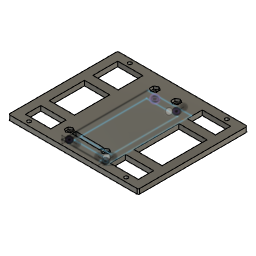
EmlaSafe - Adapter Plate (Autodesk Fusion 360 design; units mm, degrees)
Autodesk Fusion 360 part; units mm, degrees
(part 1 of 2)
sketch "Sketch1" plane through (0, 0, 0) normal (0, 0, 1) x (1, 0, 0)
  line L0 (15.5775, 37.2124) -> (15.5775, 44.1528) construction
  circle A0 centre (15.5775, 40.6826) radius 3.5
  line L1 (33.2439, 37.2427) -> (33.2439, 44.2427) construction
  circle A1 centre (33.2439, 40.7427) radius 3.5
  circle A2 centre (6.7, -23.6) radius 1.65
  circle A3 centre (42.4985, -23.8668) radius 1.65
  line L2 (6.7, -23.6) -> (6.7, -21.95) construction
  line L3 (6.7, -23.6) -> (6.7, -25.25) construction
  line L4 (42.4985, -23.8668) -> (42.4985, -22.2168) construction
  line L5 (42.4985, -23.8668) -> (42.4985, -25.5168) construction
  line L6 (42.4985, -22.2168) -> (35.9985, -22.2168)
  line L7 (35.9985, -22.2168) -> (35.9985, -25.4858)
  line L8 (35.9985, -25.4858) -> (42.4985, -25.4858)
  line L9 (42.4985, -25.4858) -> (42.4985, -22.2168)
  line L10 (6.7, -25.25) -> (13.2, -25.25)
  line L11 (13.2, -25.25) -> (13.2, -21.981)
  line L12 (13.2, -21.981) -> (6.7, -21.981)
  line L13 (6.7, -21.981) -> (6.7, -25.25)
  line L14 (50, 45) -> (50, -29)
  line L15 (50, -29) -> (1, -29)
  line L16 (1, -29) -> (1, 45)
  line L17 (13.2, -21.981) -> (35.9985, -22.2168)
  line L18 (35.9985, -25.4858) -> (13.2, -25.25)
  line L19 (50, 45) -> (50, 46.2)
  line L20 (50, 46.2) -> (1, 46.2)
  line L21 (1, 46.2) -> (1, 45)
  line L22 (8, 33) -> (8, -18)
  line L23 (43, 33) -> (43, -18)
  line L24 (43, -18) -> (8, -18)
  line L25 (8, 33) -> (43, 33)
  dimension "d1" = 7
  dimension "d2" = 7
  dimension "d3" = 3.3
  dimension "d4" = 3.3
  dimension "d5" = 6.5
  dimension "d6" = 6.5
  dimension "d7" = 49
  dimension "d8" = 74
  dimension "d15" = 1.2
  constraint vertical L0
  constraint midpoint L0 A0.centre
  constraint vertical L1
  constraint midpoint L1 A1.centre
  constraint coincident A2.centre L2.start
  constraint coincident A2 L2.end
  constraint vertical L2
  constraint coincident A2 L3.end
  constraint parallel L2 L3
  constraint coincident A3.centre L4.start
  constraint coincident A3 L4.end
  constraint vertical L4
  constraint coincident A3 L5.end
  constraint parallel L4 L5
  constraint horizontal L6
  constraint vertical L7
  constraint horizontal L8
  constraint vertical L9
  constraint horizontal L10
  constraint vertical L11
  constraint horizontal L12
  constraint vertical L13
  constraint vertical L14
  constraint horizontal L15
  constraint vertical L16
  constraint parallel L17 L18
  constraint vertical L19
  constraint horizontal L20
  constraint vertical L21
  constraint perpendicular L23 L24
  measures "d1" diameter of A1
  measures "d2" diameter of A0
  measures "d3" diameter of A2
  measures "d4" diameter of A3
  measures "d5" distance of L4.end L6.end
  measures "d6" distance of L3.end L10.end
  measures "d7" distance of L14.end L15.end
  measures "d8" distance of L14.start L14.end
  measures "d15" distance of L16.end L20.end
extrude "Extrude1" add sketch "Sketch1" along normal blind 1 contours L14 L15 L16 L19 L20 L21 | L22 L23 L24 L25 makes body 1
extrude "Extrude2" add sketch "Sketch1" along normal blind -3 and the other way blind -1 contours A0 | A1 | A2 L12 L13 | A2 L10 L11 L12 | A2 L12 L13 | A3 L6 L7 L8 | A3 L8 L9 | A3 L8 L9 bodies 1
sketch "Sketch2" plane through (0, 0, 0) normal (0, 0, 1) x (1, 0, 0)
  line L0 (79.2304, 52.3866) -> (-25.7696, 52.3866)
  line L1 (-9.7696, 51.3866) -> (63.2304, 51.3866)
  line L2 (-25.7696, -37.6134) -> (79.2304, -37.6134)
  line L3 (63.2304, -36.6134) -> (-9.7696, -36.6134)
  line L4 (-10.892, -33.3408) -> (-10.9857, -33.0965)
  line L5 (65.0576, -32.2555) -> (64.8725, -32.4405)
  line L6 (64.2304, 48.8866) -> (64.2441, 48.6253)
  line L7 (-10.9857, -33.0965) -> (-11.1045, -32.8634)
  line L8 (80.2085, -36.8213) -> (80.2304, -36.6134)
  line L9 (64.8725, -32.4405) -> (64.7079, -32.6439)
  line L10 (64.7079, -32.6439) -> (64.5653, -32.8634)
  line L11 (65.7538, -34.3283) -> (65.7304, -34.1134)
  line L12 (79.2249, -30.7179) -> (79.1814, -30.9224)
  line L13 (65.9579, 46.509) -> (66.2106, 46.4413)
  line L14 (66.1692, -33.2857) -> (66.3603, -33.1844)
  line L15 (79.2304, -30.6134) -> (79.2249, -30.7179)
  line L16 (66.4691, -31.6271) -> (66.2106, -31.668)
  line L17 (79.0964, -31.1134) -> (78.9735, -31.2825)
  line L18 (79.1814, -30.9224) -> (79.0964, -31.1134)
  line L19 (66.3603, -33.1844) -> (66.5686, -33.1265)
  line L20 (65.7304, -34.1134) -> (65.7363, -34.0052)
  line L21 (66.2106, 46.4413) -> (66.4691, 46.4003)
  line L22 (66.2106, -31.668) -> (65.9579, -31.7357)
  line L23 (79.2304, -37.6134) -> (79.3349, -37.6079)
  line L24 (67.2916, -33.2857) -> (67.3778, -33.3512)
  line L25 (67.1988, -33.2298) -> (67.2916, -33.2857)
  line L26 (-11.8001, 46.8641) -> (-11.5968, 47.0288)
  line L27 (65.9343, 48.2815) -> (65.8228, 48.4668)
  line L28 (66.083, 48.1245) -> (65.9343, 48.2815)
  line L29 (67.3778, -33.3512) -> (67.5265, -33.5082)
  line L30 (79.3349, -37.6079) -> (79.5394, -37.5644)
  line L31 (64.2304, -34.1134) -> (64.2304, -35.6134)
  line L32 (-11.5968, 47.0288) -> (-11.4117, 47.2138)
  line L33 (64.2304, -35.6134) -> (64.2085, -35.8213)
  line L34 (-12.2528, -31.8295) -> (-12.4971, -31.7357)
  line L35 (-12.0196, -31.9483) -> (-12.2528, -31.8295)
  line L36 (65.7538, 48.6717) -> (65.7304, 48.8866)
  line L37 (66.7845, -33.1148) -> (66.9979, -33.1498)
  line L38 (-12.6222, -33.3512) -> (-12.4735, -33.5082)
  line L39 (64.2441, -33.852) -> (64.2304, -34.1134)
  line L40 (66.5686, -33.1265) -> (66.7845, -33.1148)
  line L41 (66.9979, -33.1498) -> (67.1988, -33.2298)
  line L42 (78.6371, -31.5269) -> (78.4383, -31.5915)
  line L43 (78.9735, -31.2825) -> (78.8182, -31.4224)
  line L44 (65.8228, 48.4668) -> (65.7538, 48.6717)
  line L45 (-12.4971, 46.509) -> (-12.2528, 46.6028)
  line L46 (-12.362, -33.6935) -> (-12.293, -33.8984)
  line L47 (78.8182, -31.4224) -> (78.6371, -31.5269)
  line L48 (-12.2528, 46.6028) -> (-12.0196, 46.7216)
  line L49 (78.4383, -31.5915) -> (78.2304, -31.6134)
  line L50 (-12.0196, 46.7216) -> (-11.8001, 46.8641)
  line L51 (-12.4735, -33.5082) -> (-12.362, -33.6935)
  line L52 (-12.362, 48.4668) -> (-12.4735, 48.2815)
  line L53 (80.0394, -37.2011) -> (80.1439, -37.0201)
  line L54 (-11.2471, -32.6439) -> (-11.4117, -32.4405)
  line L55 (64.3528, 48.1141) -> (64.4465, 47.8698)
  line L56 (79.8995, -37.3565) -> (80.0394, -37.2011)
  line L57 (65.7136, -31.8295) -> (65.4804, -31.9483)
  line L58 (-11.4117, -32.4405) -> (-11.5968, -32.2555)
  line L59 (65.9579, -31.7357) -> (65.7136, -31.8295)
  line L60 (-12.293, 48.6717) -> (-12.362, 48.4668)
  line L61 (64.4465, 47.8698) -> (64.5653, 47.6366)
  line L62 (78.2304, -31.6134) -> (66.7304, -31.6134)
  line L63 (-24.7696, 46.3866) -> (-13.2696, 46.3866)
  line L64 (64.4465, -33.0965) -> (64.3528, -33.3408)
  line L65 (64.5653, -32.8634) -> (64.4465, -33.0965)
  line L66 (-10.7833, -33.852) -> (-10.8242, -33.5936)
  line L67 (-10.8242, -33.5936) -> (-10.892, -33.3408)
  line L68 (80.1439, -37.0201) -> (80.2085, -36.8213)
  line L69 (-12.2696, 48.8866) -> (-12.293, 48.6717)
  line L70 (64.285, 48.3669) -> (64.3528, 48.1141)
  line L71 (-12.4735, 48.2815) -> (-12.6222, 48.1245)
  line L72 (-11.1045, -32.8634) -> (-11.2471, -32.6439)
  line L73 (65.2609, -32.0908) -> (65.0576, -32.2555)
  line L74 (65.4804, -31.9483) -> (65.2609, -32.0908)
  line L75 (64.2441, 48.6253) -> (64.285, 48.3669)
  line L76 (-12.6222, 48.1245) -> (-12.7084, 48.059)
  line L77 (-13.3237, 47.8881) -> (-13.5371, 47.9231)
  line L78 (-13.8308, -33.2857) -> (-13.6397, -33.1844)
  line L79 (-13.6397, -33.1844) -> (-13.4314, -33.1265)
  line L80 (66.262, 48.0031) -> (66.083, 48.1245)
  line L81 (-10.2696, -36.4794) -> (-10.4387, -36.3565)
  line L82 (-13.4314, -33.1265) -> (-13.2155, -33.1148)
  line L83 (-12.8995, 47.9577) -> (-13.1078, 47.8998)
  line L84 (-24.8741, -31.6079) -> (-25.0786, -31.5644)
  line L85 (67.2916, -34.941) -> (67.1005, -35.0423)
  line L86 (66.4629, -35.0769) -> (66.262, -34.9969)
  line L87 (-10.0786, -36.5644) -> (-10.2696, -36.4794)
  line L88 (-13.1078, 47.8998) -> (-13.3237, 47.8881)
  line L89 (66.8922, -35.1002) -> (66.6763, -35.1119)
  line L90 (-13.2155, -33.1148) -> (-13.0021, -33.1498)
  line L91 (-13.0021, -33.1498) -> (-12.8012, -33.2298)
  line L92 (66.8922, 47.8998) -> (66.6763, 47.8881)
  line L93 (-24.7696, -31.6134) -> (-24.8741, -31.6079)
  line L94 (-13.9956, -33.4257) -> (-13.8308, -33.2857)
  line L95 (66.6763, 47.8881) -> (66.4629, 47.9231)
  line L96 (66.4629, 47.9231) -> (66.262, 48.0031)
  line L97 (-9.7696, -36.6134) -> (-9.8741, -36.6079)
  line L98 (-9.8741, -36.6079) -> (-10.0786, -36.5644)
  line L99 (67.1005, -35.0423) -> (66.8922, -35.1002)
  line L100 (-12.7084, 48.059) -> (-12.8995, 47.9577)
  line L101 (66.6763, -35.1119) -> (66.4629, -35.0769)
  line L102 (-14.2173, -33.7941) -> (-14.1265, -33.5978)
  line L103 (-12.7498, -31.668) -> (-13.0083, -31.6271)
  line L104 (67.707, 48.6717) -> (67.638, 48.4668)
  line L105 (-14.0657, 48.2815) -> (-14.1772, 48.4668)
  line L106 (66.262, -34.9969) -> (66.083, -34.8755)
  line L107 (-13.2696, -31.6134) -> (-24.7696, -31.6134)
  line L108 (-14.1265, -33.5978) -> (-13.9956, -33.4257)
  line L109 (-12.4971, -31.7357) -> (-12.7498, -31.668)
  line L110 (-13.0083, -31.6271) -> (-13.2696, -31.6134)
  line L111 (-13.917, 48.1245) -> (-14.0657, 48.2815)
  line L112 (66.7304, -31.6134) -> (66.4691, -31.6271)
  line L113 (67.7304, 48.8866) -> (67.707, 48.6717)
  line L114 (67.3778, 48.1245) -> (67.2916, 48.059)
  line L115 (67.2916, 48.059) -> (67.1005, 47.9577)
  line L116 (66.083, -34.8755) -> (65.9343, -34.7185)
  line L117 (66.4691, 46.4003) -> (66.7304, 46.3866)
  line L118 (65.8228, -34.5333) -> (65.7538, -34.3283)
  line L119 (66.7304, 46.3866) -> (78.2304, 46.3866)
  line L120 (-14.2462, 48.6717) -> (-14.2696, 48.8866)
  line L121 (67.1005, 47.9577) -> (66.8922, 47.8998)
  line L122 (-14.2637, -34.0052) -> (-14.2173, -33.7941)
  line L123 (67.5265, 48.2815) -> (67.3778, 48.1245)
  line L124 (-13.5371, 47.9231) -> (-13.738, 48.0031)
  line L125 (67.638, 48.4668) -> (67.5265, 48.2815)
  line L126 (-13.738, 48.0031) -> (-13.917, 48.1245)
  line L127 (65.9343, -34.7185) -> (65.8228, -34.5333)
  line L128 (-14.1772, 48.4668) -> (-14.2462, 48.6717)
  line L129 (-12.8995, -35.0423) -> (-13.1078, -35.1002)
  line L130 (-12.7084, -34.941) -> (-12.8995, -35.0423)
  line L131 (66.1692, 49.7143) -> (66.3603, 49.8156)
  line L132 (78.4383, 46.3648) -> (78.6371, 46.3002)
  line L133 (78.6371, 46.3002) -> (78.8182, 46.1957)
  line L134 (-10.7207, 50.6957) -> (-10.6356, 50.8866)
  line L135 (-13.1078, -35.1002) -> (-13.3237, -35.1119)
  line L136 (78.9735, 46.0558) -> (79.0964, 45.8866)
  line L137 (-13.3237, -35.1119) -> (-13.5371, -35.0769)
  line L138 (66.5686, 49.8735) -> (66.7845, 49.8852)
  line L139 (-13.5371, -35.0769) -> (-13.738, -34.9969)
  line L140 (66.7845, 49.8852) -> (66.9979, 49.8502)
  line L141 (66.3603, 49.8156) -> (66.5686, 49.8735)
  line L142 (66.0044, 49.5743) -> (66.1692, 49.7143)
  line L143 (-10.6356, 50.8866) -> (-10.5127, 51.0558)
  line L144 (-12.6222, 49.6488) -> (-12.4735, 49.4918)
  line L145 (79.1814, 45.6957) -> (79.2249, 45.4912)
  line L146 (-12.4735, 49.4918) -> (-12.362, 49.3065)
  line L147 (-12.7084, 49.7143) -> (-12.6222, 49.6488)
  line L148 (65.8735, 49.4022) -> (66.0044, 49.5743)
  line L149 (-12.293, 49.1016) -> (-12.2696, 48.8866)
  line L150 (66.9979, 49.8502) -> (67.1988, 49.7702)
  line L151 (-13.738, -34.9969) -> (-13.917, -34.8755)
  line L152 (79.2249, 45.4912) -> (79.2304, 45.3866)
  line L153 (78.8182, 46.1957) -> (78.9735, 46.0558)
  line L154 (-12.362, 49.3065) -> (-12.293, 49.1016)
  line L155 (67.1988, 49.7702) -> (67.2916, 49.7143)
  line L156 (79.0964, 45.8866) -> (79.1814, 45.6957)
  line L157 (-13.917, -34.8755) -> (-14.0657, -34.7185)
  line L158 (-12.8012, 49.7702) -> (-12.7084, 49.7143)
  line L159 (-26.7478, 51.5946) -> (-26.7696, 51.3866)
  line L160 (-10.7641, 50.4912) -> (-10.7207, 50.6957)
  line L161 (-14.0657, -34.7185) -> (-14.1772, -34.5333)
  line L162 (-14.2696, 48.8866) -> (-14.2637, 48.9948)
  line L163 (67.2916, 49.7143) -> (67.3778, 49.6488)
  line L164 (67.3778, 49.6488) -> (67.5265, 49.4918)
  line L165 (-14.1772, -34.5333) -> (-14.2462, -34.3283)
  line L166 (-13.0021, 49.8502) -> (-12.8012, 49.7702)
  line L167 (80.2304, 51.3866) -> (80.2085, 51.5946)
  line L168 (-10.7696, 48.8866) -> (-10.7696, 50.3866)
  line L169 (67.638, 49.3065) -> (67.707, 49.1016)
  line L170 (-26.2696, 52.2527) -> (-26.4387, 52.1298)
  line L171 (79.8995, 52.1298) -> (79.7304, 52.2527)
  line L172 (-13.8308, 49.7143) -> (-13.6397, 49.8156)
  line L173 (-25.7696, 45.3866) -> (-25.7478, 45.5946)
  line L174 (67.707, 49.1016) -> (67.7304, 48.8866)
  line L175 (-10.7696, 50.3866) -> (-10.7641, 50.4912)
  line L176 (80.2085, 51.5946) -> (80.1439, 51.7934)
  line L177 (-26.5786, 51.9744) -> (-26.6831, 51.7934)
  line L178 (67.5265, 49.4918) -> (67.638, 49.3065)
  line L179 (-13.2155, 49.8852) -> (-13.0021, 49.8502)
  line L180 (-26.4387, 52.1298) -> (-26.5786, 51.9744)
  line L181 (80.0394, 51.9744) -> (79.8995, 52.1298)
  line L182 (-13.6397, 49.8156) -> (-13.4314, 49.8735)
  line L183 (80.1439, 51.7934) -> (80.0394, 51.9744)
  line L184 (-26.6831, 51.7934) -> (-26.7478, 51.5946)
  line L185 (-13.4314, 49.8735) -> (-13.2155, 49.8852)
  line L186 (-14.2462, -34.3283) -> (-14.2696, -34.1134)
  line L187 (79.3349, 52.3812) -> (79.2304, 52.3866)
  line L188 (-10.8242, 48.3669) -> (-10.7833, 48.6253)
  line L189 (64.7079, 47.4172) -> (64.8725, 47.2138)
  line L190 (63.3349, -36.6079) -> (63.2304, -36.6134)
  line L191 (-10.7833, 48.6253) -> (-10.7696, 48.8866)
  line L192 (64.5653, 47.6366) -> (64.7079, 47.4172)
  line L193 (-10.7696, -35.6134) -> (-10.7696, -34.1134)
  line L194 (-12.7498, 46.4413) -> (-12.4971, 46.509)
  line L195 (67.638, -34.5333) -> (67.5265, -34.7185)
  line L196 (67.7304, -34.1134) -> (67.707, -34.3283)
  line L197 (-25.0786, -31.5644) -> (-25.2696, -31.4794)
  line L198 (-10.4387, -36.3565) -> (-10.5786, -36.2011)
  line L199 (63.4383, 51.3648) -> (63.6371, 51.3002)
  line L200 (-25.5786, -31.2011) -> (-25.6831, -31.0201)
  line L201 (67.3778, -34.8755) -> (67.2916, -34.941)
  line L202 (-10.7696, -34.1134) -> (-10.7833, -33.852)
  line L203 (-25.7478, -30.8213) -> (-25.7696, -30.6134)
  line L204 (63.9735, 51.0558) -> (64.0964, 50.8866)
  line L205 (-26.0786, -37.5644) -> (-25.8741, -37.6079)
  line L206 (-12.8012, -33.2298) -> (-12.7084, -33.2857)
  line L207 (-13.2696, 46.3866) -> (-13.0083, 46.4003)
  line L208 (-13.0083, 46.4003) -> (-12.7498, 46.4413)
  line L209 (67.5265, -34.7185) -> (67.3778, -34.8755)
  line L210 (-25.8741, -37.6079) -> (-25.7696, -37.6134)
  line L211 (67.707, -34.3283) -> (67.638, -34.5333)
  line L212 (-25.2696, -31.4794) -> (-25.4387, -31.3565)
  line L213 (63.2304, 51.3866) -> (63.4383, 51.3648)
  line L214 (-10.5786, -36.2011) -> (-10.6831, -36.0201)
  line L215 (-25.4387, -31.3565) -> (-25.5786, -31.2011)
  line L216 (-10.6831, -36.0201) -> (-10.7478, -35.8213)
  line L217 (63.6371, 51.3002) -> (63.8182, 51.1957)
  line L218 (-10.7478, -35.8213) -> (-10.7696, -35.6134)
  line L219 (63.8182, 51.1957) -> (63.9735, 51.0558)
  line L220 (-12.7084, -33.2857) -> (-12.6222, -33.3512)
  line L221 (-25.6831, -31.0201) -> (-25.7478, -30.8213)
  line L222 (63.7304, -36.4794) -> (63.5394, -36.5644)
  line L223 (79.7304, -37.4794) -> (79.8995, -37.3565)
  line L224 (63.5394, -36.5644) -> (63.3349, -36.6079)
  line L225 (63.8995, -36.3565) -> (63.7304, -36.4794)
  line L226 (-10.892, 48.1141) -> (-10.8242, 48.3669)
  line L227 (64.8725, 47.2138) -> (65.0576, 47.0288)
  line L228 (-10.9857, 47.8698) -> (-10.892, 48.1141)
  line L229 (65.0576, 47.0288) -> (65.2609, 46.8641)
  line L230 (66.0044, -33.4257) -> (66.1692, -33.2857)
  line L231 (64.1439, -36.0201) -> (64.0394, -36.2011)
  line L232 (-11.5968, -32.2555) -> (-11.8001, -32.0908)
  line L233 (64.0394, -36.2011) -> (63.8995, -36.3565)
  line L234 (65.4804, 46.7216) -> (65.7136, 46.6028)
  line L235 (67.638, -33.6935) -> (67.707, -33.8984)
  line L236 (-11.1045, 47.6366) -> (-10.9857, 47.8698)
  line L237 (-11.4117, 47.2138) -> (-11.2471, 47.4172)
  line L238 (65.2609, 46.8641) -> (65.4804, 46.7216)
  line L239 (79.5394, -37.5644) -> (79.7304, -37.4794)
  line L240 (65.7136, 46.6028) -> (65.9579, 46.509)
  line L241 (67.5265, -33.5082) -> (67.638, -33.6935)
  line L242 (64.2085, -35.8213) -> (64.1439, -36.0201)
  line L243 (-11.2471, 47.4172) -> (-11.1045, 47.6366)
  line L244 (-11.8001, -32.0908) -> (-12.0196, -31.9483)
  line L245 (80.2304, -36.6134) -> (80.2304, 51.3866)
  line L246 (79.2304, 7.3866) -> (79.2304, -30.6134)
  line L247 (79.2304, 45.3866) -> (79.2304, 7.3866)
  line L248 (64.285, -33.5936) -> (64.2441, -33.852)
  line L249 (64.3528, -33.3408) -> (64.285, -33.5936)
  line L250 (65.7827, -33.7941) -> (65.8735, -33.5978)
  line L251 (65.8735, -33.5978) -> (66.0044, -33.4257)
  line L252 (-26.7696, 51.3866) -> (-26.7696, -36.6134)
  line L253 (-25.7696, -30.6134) -> (-25.7696, 45.3866)
  line L254 (65.7363, -34.0052) -> (65.7827, -33.7941)
  line L255 (-25.7696, 52.3866) -> (-25.8741, 52.3812)
  line L256 (-25.4387, 46.1298) -> (-25.2696, 46.2527)
  line L257 (-13.9956, 49.5743) -> (-13.8308, 49.7143)
  line L258 (-14.1265, 49.4022) -> (-13.9956, 49.5743)
  line L259 (-25.5786, 45.9744) -> (-25.4387, 46.1298)
  line L260 (-26.0786, 52.3377) -> (-26.2696, 52.2527)
  line L261 (-14.2637, 48.9948) -> (-14.2173, 49.2059)
  line L262 (-25.0786, 46.3377) -> (-24.8741, 46.3812)
  line L263 (-25.2696, 46.2527) -> (-25.0786, 46.3377)
  line L264 (-25.7478, 45.5946) -> (-25.6831, 45.7934)
  line L265 (-24.8741, 46.3812) -> (-24.7696, 46.3866)
  line L266 (79.7304, 52.2527) -> (79.5394, 52.3377)
  line L267 (-14.2173, 49.2059) -> (-14.1265, 49.4022)
  line L268 (-25.8741, 52.3812) -> (-26.0786, 52.3377)
  line L269 (79.5394, 52.3377) -> (79.3349, 52.3812)
  line L270 (-25.6831, 45.7934) -> (-25.5786, 45.9744)
  line L271 (-26.7478, -36.8213) -> (-26.6831, -37.0201)
  line L272 (-10.5127, 51.0558) -> (-10.3574, 51.1957)
  line L273 (65.7827, 49.2059) -> (65.8735, 49.4022)
  line L274 (-26.2696, -37.4794) -> (-26.0786, -37.5644)
  line L275 (-10.3574, 51.1957) -> (-10.1763, 51.3002)
  line L276 (-12.293, -34.3283) -> (-12.362, -34.5333)
  line L277 (-12.293, -33.8984) -> (-12.2696, -34.1134)
  line L278 (-26.4387, -37.3565) -> (-26.2696, -37.4794)
  line L279 (64.2249, 50.4912) -> (64.2304, 50.3866)
  line L280 (64.2304, 50.3866) -> (64.2304, 48.8866)
  line L281 (-26.5786, -37.2011) -> (-26.4387, -37.3565)
  line L282 (64.0964, 50.8866) -> (64.1815, 50.6957)
  line L283 (-9.9775, 51.3648) -> (-9.7696, 51.3866)
  line L284 (-26.6831, -37.0201) -> (-26.5786, -37.2011)
  line L285 (65.7363, 48.9948) -> (65.7827, 49.2059)
  line L286 (78.2304, 46.3866) -> (78.4383, 46.3648)
  line L287 (-14.2696, -34.1134) -> (-14.2637, -34.0052)
  line L288 (-10.1763, 51.3002) -> (-9.9775, 51.3648)
  line L289 (-26.7696, -36.6134) -> (-26.7478, -36.8213)
  line L290 (67.707, -33.8984) -> (67.7304, -34.1134)
  line L291 (-12.4735, -34.7185) -> (-12.6222, -34.8755)
  line L292 (64.1815, 50.6957) -> (64.2249, 50.4912)
  line L293 (-12.2696, -34.1134) -> (-12.293, -34.3283)
  line L294 (-12.362, -34.5333) -> (-12.4735, -34.7185)
  line L295 (65.7304, 48.8866) -> (65.7363, 48.9948)
  line L296 (-12.6222, -34.8755) -> (-12.7084, -34.941)
  line L297 (79.2304, 52.3866) -> (79.3349, 52.3812)
  line L298 (-25.7696, 52.3866) -> (79.2304, 52.3866)
  line L299 (79.3349, 52.3812) -> (79.5394, 52.3377)
  line L300 (80.0394, 51.9744) -> (80.1439, 51.7934)
  line L301 (79.3349, -37.6079) -> (79.2304, -37.6134)
  line L302 (79.5394, 52.3377) -> (79.7304, 52.2527)
  line L303 (79.8995, 52.1298) -> (80.0394, 51.9744)
  line L304 (-26.7696, -36.6134) -> (-26.7696, 51.3866)
  line L305 (79.5394, -37.5644) -> (79.3349, -37.6079)
  line L306 (79.8995, -37.3565) -> (79.7304, -37.4794)
  line L307 (-26.6831, -37.0201) -> (-26.7478, -36.8213)
  line L308 (79.7304, -37.4794) -> (79.5394, -37.5644)
  line L309 (80.1439, -37.0201) -> (80.0394, -37.2011)
  line L310 (80.2304, -36.6134) -> (80.2085, -36.8213)
  line L311 (80.2304, 51.3866) -> (80.2304, -36.6134)
  line L312 (80.0394, -37.2011) -> (79.8995, -37.3565)
  line L313 (-26.7696, 51.3866) -> (-26.7478, 51.5946)
  line L314 (80.1439, 51.7934) -> (80.2085, 51.5946)
  line L315 (79.2304, -37.6134) -> (-25.7696, -37.6134)
  line L316 (-25.8741, -37.6079) -> (-26.0786, -37.5644)
  line L317 (-25.7696, -37.6134) -> (-25.8741, -37.6079)
  line L318 (-26.2696, -37.4794) -> (-26.4387, -37.3565)
  line L319 (79.7304, 52.2527) -> (79.8995, 52.1298)
  line L320 (-26.7478, -36.8213) -> (-26.7696, -36.6134)
  line L321 (-26.0786, -37.5644) -> (-26.2696, -37.4794)
  line L322 (80.2085, -36.8213) -> (80.1439, -37.0201)
  line L323 (-13.2696, -31.6134) -> (-13.0083, -31.6271)
  line L324 (-9.7696, 51.3866) -> (-9.9775, 51.3648)
  line L325 (-10.7833, 48.6253) -> (-10.8242, 48.3669)
  line L326 (-10.7641, 50.4912) -> (-10.7696, 50.3866)
  line L327 (-25.2696, 46.2527) -> (-25.4387, 46.1298)
  line L328 (-11.8001, -32.0908) -> (-11.5968, -32.2555)
  line L329 (-25.4387, 46.1298) -> (-25.5786, 45.9744)
  line L330 (-25.0786, 46.3377) -> (-25.2696, 46.2527)
  line L331 (-9.9775, 51.3648) -> (-10.1763, 51.3002)
  line L332 (-10.5127, 51.0558) -> (-10.6356, 50.8866)
  line L333 (-25.7696, -30.6134) -> (-25.7478, -30.8213)
  line L334 (-25.5786, 45.9744) -> (-25.6831, 45.7934)
  line L335 (-11.5968, -32.2555) -> (-11.4117, -32.4405)
  line L336 (-11.2471, 47.4172) -> (-11.4117, 47.2138)
  line L337 (-11.4117, 47.2138) -> (-11.5968, 47.0288)
  line L338 (-12.0196, 46.7216) -> (-12.2528, 46.6028)
  line L339 (-10.6356, 50.8866) -> (-10.7207, 50.6957)
  line L340 (-13.0083, -31.6271) -> (-12.7498, -31.668)
  line L341 (-26.7478, 51.5946) -> (-26.6831, 51.7934)
  line L342 (-25.7478, -30.8213) -> (-25.6831, -31.0201)
  line L343 (-10.7696, 48.8866) -> (-10.7833, 48.6253)
  line L344 (-13.2696, 46.3866) -> (-24.7696, 46.3866)
  line L345 (-25.5786, -31.2011) -> (-25.4387, -31.3565)
  line L346 (-11.5968, 47.0288) -> (-11.8001, 46.8641)
  line L347 (-11.1045, 47.6366) -> (-11.2471, 47.4172)
  line L348 (-10.892, 48.1141) -> (-10.9857, 47.8698)
  line L349 (-12.2528, 46.6028) -> (-12.4971, 46.509)
  line L350 (-11.8001, 46.8641) -> (-12.0196, 46.7216)
  line L351 (-12.7498, -31.668) -> (-12.4971, -31.7357)
  line L352 (-26.5786, -37.2011) -> (-26.6831, -37.0201)
  line L353 (-12.0196, -31.9483) -> (-11.8001, -32.0908)
  line L354 (-10.7696, 50.3866) -> (-10.7696, 48.8866)
  line L355 (-11.2471, -32.6439) -> (-11.1045, -32.8634)
  line L356 (-11.4117, -32.4405) -> (-11.2471, -32.6439)
  line L357 (-26.6831, 51.7934) -> (-26.5786, 51.9744)
  line L358 (-25.7478, 45.5946) -> (-25.7696, 45.3866)
  line L359 (-25.2696, -31.4794) -> (-25.0786, -31.5644)
  line L360 (-26.0786, 52.3377) -> (-25.8741, 52.3812)
  line L361 (-10.3574, 51.1957) -> (-10.5127, 51.0558)
  line L362 (-25.6831, -31.0201) -> (-25.5786, -31.2011)
  line L363 (-12.7498, 46.4413) -> (-13.0083, 46.4003)
  line L364 (-12.4971, 46.509) -> (-12.7498, 46.4413)
  line L365 (-25.0786, -31.5644) -> (-24.8741, -31.6079)
  line L366 (-13.0083, 46.4003) -> (-13.2696, 46.3866)
  line L367 (63.2304, 51.3866) -> (-9.7696, 51.3866)
  line L368 (-10.9857, -33.0965) -> (-10.892, -33.3408)
  line L369 (-26.4387, -37.3565) -> (-26.5786, -37.2011)
  line L370 (-26.2696, 52.2527) -> (-26.0786, 52.3377)
  line L371 (80.2085, 51.5946) -> (80.2304, 51.3866)
  line L372 (-25.7696, 45.3866) -> (-25.7696, -30.6134)
  line L373 (-10.8242, 48.3669) -> (-10.892, 48.1141)
  line L374 (-25.8741, 52.3812) -> (-25.7696, 52.3866)
  line L375 (-24.7696, 46.3866) -> (-24.8741, 46.3812)
  line L376 (-24.8741, 46.3812) -> (-25.0786, 46.3377)
  line L377 (-25.6831, 45.7934) -> (-25.7478, 45.5946)
  line L378 (78.8182, 46.1957) -> (78.6371, 46.3002)
  line L379 (-26.4387, 52.1298) -> (-26.2696, 52.2527)
  line L380 (-24.8741, -31.6079) -> (-24.7696, -31.6134)
  line L381 (-9.7696, -36.6134) -> (63.2304, -36.6134)
  line L382 (63.5394, -36.5644) -> (63.7304, -36.4794)
  line L383 (64.5653, -32.8634) -> (64.7079, -32.6439)
  line L384 (64.2304, -35.6134) -> (64.2304, -34.1134)
  line L385 (64.2304, -34.1134) -> (64.2441, -33.852)
  line L386 (-10.6831, -36.0201) -> (-10.5786, -36.2011)
  line L387 (78.9735, -31.2825) -> (79.0964, -31.1134)
  line L388 (-9.8741, -36.6079) -> (-9.7696, -36.6134)
  line L389 (79.0964, 45.8866) -> (78.9735, 46.0558)
  line L390 (-10.2696, -36.4794) -> (-10.0786, -36.5644)
  line L391 (-10.8242, -33.5936) -> (-10.7833, -33.852)
  line L392 (64.1439, -36.0201) -> (64.2085, -35.8213)
  line L393 (78.2304, -31.6134) -> (78.4383, -31.5915)
  line L394 (66.2106, 46.4413) -> (65.9579, 46.509)
  line L395 (-10.7207, 50.6957) -> (-10.7641, 50.4912)
  line L396 (64.285, -33.5936) -> (64.3528, -33.3408)
  line L397 (65.7136, -31.8295) -> (65.9579, -31.7357)
  line L398 (78.4383, -31.5915) -> (78.6371, -31.5269)
  line L399 (64.2441, -33.852) -> (64.285, -33.5936)
  line L400 (-10.4387, -36.3565) -> (-10.2696, -36.4794)
  line L401 (64.3528, -33.3408) -> (64.4465, -33.0965)
  line L402 (65.4804, -31.9483) -> (65.7136, -31.8295)
  line L403 (63.3349, -36.6079) -> (63.5394, -36.5644)
  line L404 (-10.7833, -33.852) -> (-10.7696, -34.1134)
  line L405 (65.7136, 46.6028) -> (65.4804, 46.7216)
  line L406 (-11.1045, -32.8634) -> (-10.9857, -33.0965)
  line L407 (78.6371, 46.3002) -> (78.4383, 46.3648)
  line L408 (63.8995, -36.3565) -> (64.0394, -36.2011)
  line L409 (78.8182, -31.4224) -> (78.9735, -31.2825)
  line L410 (65.2609, 46.8641) -> (65.0576, 47.0288)
  line L411 (78.6371, -31.5269) -> (78.8182, -31.4224)
  line L412 (-10.7478, -35.8213) -> (-10.6831, -36.0201)
  line L413 (-10.1763, 51.3002) -> (-10.3574, 51.1957)
  line L414 (66.7304, -31.6134) -> (78.2304, -31.6134)
  line L415 (65.2609, -32.0908) -> (65.4804, -31.9483)
  line L416 (-25.4387, -31.3565) -> (-25.2696, -31.4794)
  line L417 (66.2106, -31.668) -> (66.4691, -31.6271)
  line L418 (79.2304, -30.6134) -> (79.2304, 7.3866)
  line L419 (64.7079, -32.6439) -> (64.8725, -32.4405)
  line L420 (79.0964, -31.1134) -> (79.1814, -30.9224)
  line L421 (-10.9857, 47.8698) -> (-11.1045, 47.6366)
  line L422 (79.2249, 45.4912) -> (79.1814, 45.6957)
  line L423 (-24.7696, -31.6134) -> (-13.2696, -31.6134)
  line L424 (78.4383, 46.3648) -> (78.2304, 46.3866)
  line L425 (-10.892, -33.3408) -> (-10.8242, -33.5936)
  line L426 (64.8725, -32.4405) -> (65.0576, -32.2555)
  line L427 (-10.0786, -36.5644) -> (-9.8741, -36.6079)
  line L428 (66.4691, 46.4003) -> (66.2106, 46.4413)
  line L429 (65.4804, 46.7216) -> (65.2609, 46.8641)
  line L430 (78.2304, 46.3866) -> (66.7304, 46.3866)
  line L431 (-26.5786, 51.9744) -> (-26.4387, 52.1298)
  line L432 (66.7304, 46.3866) -> (66.4691, 46.4003)
  line L433 (66.4691, -31.6271) -> (66.7304, -31.6134)
  line L434 (63.2304, -36.6134) -> (63.3349, -36.6079)
  line L435 (63.7304, -36.4794) -> (63.8995, -36.3565)
  line L436 (65.0576, 47.0288) -> (64.8725, 47.2138)
  line L437 (-12.4971, -31.7357) -> (-12.2528, -31.8295)
  line L438 (65.9579, 46.509) -> (65.7136, 46.6028)
  line L439 (64.2085, -35.8213) -> (64.2304, -35.6134)
  line L440 (79.2249, -30.7179) -> (79.2304, -30.6134)
  line L441 (-12.2528, -31.8295) -> (-12.0196, -31.9483)
  line L442 (67.707, 49.1016) -> (67.638, 49.3065)
  line L443 (66.9979, -33.1498) -> (66.7845, -33.1148)
  line L444 (67.1005, -35.0423) -> (67.2916, -34.941)
  line L445 (65.7538, -34.3283) -> (65.8228, -34.5333)
  line L446 (64.2304, 50.3866) -> (64.2249, 50.4912)
  line L447 (66.4629, -35.0769) -> (66.6763, -35.1119)
  line L448 (65.7827, -33.7941) -> (65.7363, -34.0052)
  line L449 (66.1692, -33.2857) -> (66.0044, -33.4257)
  line L450 (64.2304, 48.8866) -> (64.2304, 50.3866)
  line L451 (79.1814, 45.6957) -> (79.0964, 45.8866)
  line L452 (67.707, -33.8984) -> (67.638, -33.6935)
  line L453 (64.0394, -36.2011) -> (64.1439, -36.0201)
  line L454 (79.2304, 45.3866) -> (79.2249, 45.4912)
  line L455 (66.6763, -35.1119) -> (66.8922, -35.1002)
  line L456 (64.7079, 47.4172) -> (64.5653, 47.6366)
  line L457 (67.2916, -34.941) -> (67.3778, -34.8755)
  line L458 (67.7304, 48.8866) -> (67.707, 49.1016)
  line L459 (79.2304, 7.3866) -> (79.2304, 45.3866)
  line L460 (-10.7696, -35.6134) -> (-10.7478, -35.8213)
  line L461 (67.638, -33.6935) -> (67.5265, -33.5082)
  line L462 (67.707, 48.6717) -> (67.7304, 48.8866)
  line L463 (67.2916, -33.2857) -> (67.1988, -33.2298)
  line L464 (65.8228, -34.5333) -> (65.9343, -34.7185)
  line L465 (64.3528, 48.1141) -> (64.285, 48.3669)
  line L466 (66.083, 48.1245) -> (66.262, 48.0031)
  line L467 (66.4629, 47.9231) -> (66.6763, 47.8881)
  line L468 (67.3778, -34.8755) -> (67.5265, -34.7185)
  line L469 (64.2441, 48.6253) -> (64.2304, 48.8866)
  line L470 (67.3778, 48.1245) -> (67.5265, 48.2815)
  line L471 (67.5265, -33.5082) -> (67.3778, -33.3512)
  line L472 (63.8182, 51.1957) -> (63.6371, 51.3002)
  line L473 (67.638, 49.3065) -> (67.5265, 49.4918)
  line L474 (66.262, -34.9969) -> (66.4629, -35.0769)
  line L475 (64.8725, 47.2138) -> (64.7079, 47.4172)
  line L476 (63.9735, 51.0558) -> (63.8182, 51.1957)
  line L477 (66.083, -34.8755) -> (66.262, -34.9969)
  line L478 (-10.5786, -36.2011) -> (-10.4387, -36.3565)
  line L479 (65.9343, 48.2815) -> (66.083, 48.1245)
  line L480 (67.1988, -33.2298) -> (66.9979, -33.1498)
  line L481 (65.7363, -34.0052) -> (65.7304, -34.1134)
  line L482 (64.1815, 50.6957) -> (64.0964, 50.8866)
  line L483 (67.3778, -33.3512) -> (67.2916, -33.2857)
  line L484 (64.0964, 50.8866) -> (63.9735, 51.0558)
  line L485 (78.9735, 46.0558) -> (78.8182, 46.1957)
  line L486 (64.5653, 47.6366) -> (64.4465, 47.8698)
  line L487 (-10.7696, -34.1134) -> (-10.7696, -35.6134)
  line L488 (67.7304, -34.1134) -> (67.707, -33.8984)
  line L489 (66.0044, -33.4257) -> (65.8735, -33.5978)
  line L490 (65.9579, -31.7357) -> (66.2106, -31.668)
  line L491 (63.6371, 51.3002) -> (63.4383, 51.3648)
  line L492 (66.6763, 47.8881) -> (66.8922, 47.8998)
  line L493 (67.5265, -34.7185) -> (67.638, -34.5333)
  line L494 (67.638, 48.4668) -> (67.707, 48.6717)
  line L495 (64.2249, 50.4912) -> (64.1815, 50.6957)
  line L496 (79.1814, -30.9224) -> (79.2249, -30.7179)
  line L497 (67.5265, 48.2815) -> (67.638, 48.4668)
  line L498 (65.0576, -32.2555) -> (65.2609, -32.0908)
  line L499 (65.9343, -34.7185) -> (66.083, -34.8755)
  line L500 (64.285, 48.3669) -> (64.2441, 48.6253)
  line L501 (67.1005, 47.9577) -> (67.2916, 48.059)
  line L502 (67.5265, 49.4918) -> (67.3778, 49.6488)
  line L503 (66.8922, -35.1002) -> (67.1005, -35.0423)
  line L504 (65.7304, -34.1134) -> (65.7538, -34.3283)
  line L505 (64.4465, -33.0965) -> (64.5653, -32.8634)
  line L506 (-13.2155, 49.8852) -> (-13.4314, 49.8735)
  line L507 (-14.0657, -34.7185) -> (-13.917, -34.8755)
  line L508 (-12.4735, 49.4918) -> (-12.6222, 49.6488)
  line L509 (-13.6397, 49.8156) -> (-13.8308, 49.7143)
  line L510 (-12.293, 48.6717) -> (-12.2696, 48.8866)
  line L511 (65.7304, 48.8866) -> (65.7538, 48.6717)
  line L512 (-14.1265, -33.5978) -> (-14.2173, -33.7941)
  line L513 (-12.362, -33.6935) -> (-12.4735, -33.5082)
  line L514 (67.2916, 49.7143) -> (67.1988, 49.7702)
  line L515 (-13.2155, -33.1148) -> (-13.4314, -33.1265)
  line L516 (-14.2696, -34.1134) -> (-14.2462, -34.3283)
  line L517 (-13.0021, -33.1498) -> (-13.2155, -33.1148)
  line L518 (66.262, 48.0031) -> (66.4629, 47.9231)
  line L519 (-13.6397, -33.1844) -> (-13.8308, -33.2857)
  line L520 (66.3603, 49.8156) -> (66.1692, 49.7143)
  line L521 (-13.4314, -33.1265) -> (-13.6397, -33.1844)
  line L522 (-13.917, -34.8755) -> (-13.738, -34.9969)
  line L523 (67.3778, 49.6488) -> (67.2916, 49.7143)
  line L524 (-12.293, -34.3283) -> (-12.2696, -34.1134)
  line L525 (-12.2696, 48.8866) -> (-12.293, 49.1016)
  line L526 (-12.7084, -34.941) -> (-12.6222, -34.8755)
  line L527 (-12.7084, -33.2857) -> (-12.8012, -33.2298)
  line L528 (66.5686, 49.8735) -> (66.3603, 49.8156)
  line L529 (-14.2462, -34.3283) -> (-14.1772, -34.5333)
  line L530 (-12.4735, 48.2815) -> (-12.362, 48.4668)
  line L531 (67.707, -34.3283) -> (67.7304, -34.1134)
  line L532 (65.7538, 48.6717) -> (65.8228, 48.4668)
  line L533 (66.3603, -33.1844) -> (66.1692, -33.2857)
  line L534 (-14.2637, -34.0052) -> (-14.2696, -34.1134)
  line L535 (65.7363, 48.9948) -> (65.7304, 48.8866)
  line L536 (-14.2173, -33.7941) -> (-14.2637, -34.0052)
  line L537 (-13.8308, -33.2857) -> (-13.9956, -33.4257)
  line L538 (-12.6222, -34.8755) -> (-12.4735, -34.7185)
  line L539 (67.638, -34.5333) -> (67.707, -34.3283)
  line L540 (65.7827, 49.2059) -> (65.7363, 48.9948)
  line L541 (-12.2696, -34.1134) -> (-12.293, -33.8984)
  line L542 (-13.9956, 49.5743) -> (-14.1265, 49.4022)
  line L543 (-13.738, -34.9969) -> (-13.5371, -35.0769)
  line L544 (66.0044, 49.5743) -> (65.8735, 49.4022)
  line L545 (-12.4735, -33.5082) -> (-12.6222, -33.3512)
  line L546 (-12.7084, 49.7143) -> (-12.8012, 49.7702)
  line L547 (-14.1265, 49.4022) -> (-14.2173, 49.2059)
  line L548 (66.7845, 49.8852) -> (66.5686, 49.8735)
  line L549 (-14.1772, -34.5333) -> (-14.0657, -34.7185)
  line L550 (-12.362, 48.4668) -> (-12.293, 48.6717)
  line L551 (-13.8308, 49.7143) -> (-13.9956, 49.5743)
  line L552 (65.8735, -33.5978) -> (65.7827, -33.7941)
  line L553 (-14.2173, 49.2059) -> (-14.2637, 48.9948)
  line L554 (-14.2637, 48.9948) -> (-14.2696, 48.8866)
  line L555 (-13.4314, 49.8735) -> (-13.6397, 49.8156)
  line L556 (-13.9956, -33.4257) -> (-14.1265, -33.5978)
  line L557 (66.8922, 47.8998) -> (67.1005, 47.9577)
  line L558 (-12.8012, -33.2298) -> (-13.0021, -33.1498)
  line L559 (-12.8012, 49.7702) -> (-13.0021, 49.8502)
  line L560 (66.5686, -33.1265) -> (66.3603, -33.1844)
  line L561 (65.8735, 49.4022) -> (65.7827, 49.2059)
  line L562 (-12.8995, -35.0423) -> (-12.7084, -34.941)
  line L563 (65.8228, 48.4668) -> (65.9343, 48.2815)
  line L564 (66.7845, -33.1148) -> (66.5686, -33.1265)
  line L565 (-13.0021, 49.8502) -> (-13.2155, 49.8852)
  line L566 (64.4465, 47.8698) -> (64.3528, 48.1141)
  line L567 (63.4383, 51.3648) -> (63.2304, 51.3866)
  line L568 (67.2916, 48.059) -> (67.3778, 48.1245)
  line L569 (-12.362, -34.5333) -> (-12.293, -34.3283)
  line L570 (66.1692, 49.7143) -> (66.0044, 49.5743)
  line L571 (-13.3237, 47.8881) -> (-13.1078, 47.8998)
  line L572 (-14.1772, 48.4668) -> (-14.0657, 48.2815)
  line L573 (-13.917, 48.1245) -> (-13.738, 48.0031)
  line L574 (-14.0657, 48.2815) -> (-13.917, 48.1245)
  line L575 (-12.7084, 48.059) -> (-12.6222, 48.1245)
  line L576 (-12.6222, 48.1245) -> (-12.4735, 48.2815)
  line L577 (-12.8995, 47.9577) -> (-12.7084, 48.059)
  line L578 (-12.293, 49.1016) -> (-12.362, 49.3065)
  line L579 (-13.738, 48.0031) -> (-13.5371, 47.9231)
  line L580 (-12.362, 49.3065) -> (-12.4735, 49.4918)
  line L581 (-13.3237, -35.1119) -> (-13.1078, -35.1002)
  line L582 (67.1988, 49.7702) -> (66.9979, 49.8502)
  line L583 (-12.6222, 49.6488) -> (-12.7084, 49.7143)
  line L584 (-13.5371, -35.0769) -> (-13.3237, -35.1119)
  line L585 (-12.4735, -34.7185) -> (-12.362, -34.5333)
  line L586 (-13.5371, 47.9231) -> (-13.3237, 47.8881)
  line L587 (-14.2462, 48.6717) -> (-14.1772, 48.4668)
  line L588 (-13.1078, 47.8998) -> (-12.8995, 47.9577)
  line L589 (-13.1078, -35.1002) -> (-12.8995, -35.0423)
  line L590 (-14.2696, 48.8866) -> (-14.2462, 48.6717)
  line L591 (66.9979, 49.8502) -> (66.7845, 49.8852)
  line L592 (-12.293, -33.8984) -> (-12.362, -33.6935)
  line L593 (-12.6222, -33.3512) -> (-12.7084, -33.2857)
  point P0 (26.7304, 7.3866)
sketch "Sketch3" plane through (0, 0, 0) normal (0, 0, 1) x (1, 0, 0)
  circle A0 centre (66.7314, -34.1104) radius 1.5
  circle A1 centre (-13.2753, -34.1171) radius 1.5
  circle A2 centre (-13.2624, 48.8983) radius 1.5
  circle A3 centre (66.7239, 48.8933) radius 1.5
  line L0 (73.2304, 45.3866) -> (-19.7696, 45.3866)
  line L1 (-19.7696, 45.3866) -> (-19.7696, -30.587)
  line L2 (-19.7696, -30.587) -> (73.2304, -30.587)
  line L3 (73.2304, -30.587) -> (73.2304, 45.3866)
  line L4 (1, -29) -> (50, -29)
  line L5 (50, -29) -> (50, -30.587)
  line L6 (50, -30.587) -> (1, -30.587)
  line L7 (1, -30.587) -> (1, -29)
  line L8 (1, 25) -> (-19.7696, 25)
  line L9 (-19.7696, 25) -> (-19.7696, 18)
  line L10 (-19.7696, 18) -> (1, 18)
  line L11 (1, 18) -> (1, 25)
  line L12 (1, -29) -> (1, 45)
  line L13 (73.2304, 33) -> (73.2304, 26)
  line L14 (50, -18) -> (73.2304, -18)
  line L15 (73.2304, -18) -> (73.2304, -11)
  line L16 (73.2304, -11) -> (50, -11)
  line L17 (50, -11) -> (50, -18)
  line L18 (50, 45) -> (50, -29)
  line L19 (1, -18) -> (-19.7696, -18)
  line L20 (-19.7696, -18) -> (-19.7696, -11)
  line L21 (-19.7696, -11) -> (1, -11)
  line L22 (1, -11) -> (1, -18)
  line L23 (73.2304, 33) -> (50, 33)
  line L24 (50, 33) -> (50, 26)
  line L25 (50, 26) -> (73.2304, 26)
  line L26 (73.2304, 26) -> (73.2304, 33)
  line L27 (-26.7696, 52.3866) -> (80.2313, 52.3866)
  line L28 (80.2313, 52.3866) -> (80.2313, -37.6134)
  line L29 (80.2313, -37.6134) -> (-26.7696, -37.6134)
  line L30 (-26.7696, -37.6134) -> (-26.7696, 52.3866)
  point P0 (66.7314, -34.1104)
  point P1 (-13.2753, -34.1171)
  point P2 (-13.2624, 48.8983)
  point P3 (66.7239, 48.8933)
  point P4 (1, -29)
  point P5 (-26.7696, 52.3866)
  point P6 (80.2313, -37.6134)
  dimension "d19" = 3
  dimension "d21" = 3
  dimension "d23" = 3
  dimension "d25" = 3
  dimension "d30" = 7
  dimension "d32" = 7
  dimension "d33" = 7
  constraint coincident P0 A0.centre
  constraint coincident P1 A1.centre
  constraint coincident P2 A2.centre
  constraint coincident P3 A3.centre
  constraint horizontal L0
  constraint vertical L1
  constraint horizontal L2
  constraint vertical L3
  constraint horizontal L4
  constraint vertical L5
  constraint horizontal L6
  constraint vertical L7
  constraint coincident L2 L5.end
  constraint coincident P4 L4.start
  constraint horizontal L8
  constraint vertical L9
  constraint horizontal L10
  constraint vertical L11
  constraint coincident L1 L9.end
  constraint coincident L8.start L12
  constraint vertical L13
  constraint horizontal L14
  constraint vertical L15
  constraint horizontal L16
  constraint vertical L17
  constraint coincident L14.start L18
  constraint horizontal L19
  constraint vertical L20
  constraint horizontal L21
  constraint vertical L22
  constraint coincident L12 L19.start
  constraint horizontal L23
  constraint vertical L24
  constraint horizontal L25
  constraint vertical L26
  constraint coincident L18 L24.end
  constraint horizontal L27
  constraint vertical L28
  constraint horizontal L29
  constraint vertical L30
  constraint coincident P6 L28.end
  constraint coincident P5 L27.start
  measures "d19" diameter of A0
  measures "d21" diameter of A1
  measures "d23" diameter of A2
  measures "d25" diameter of A3
  measures "d30" distance of L8.start L10.end
  measures "d32" distance of L14.start L16.end
  measures "d33" distance of L19.start L21.end
extrude "Extrude3" add sketch "Sketch3" along normal blind 1 contours L3 L13 L18 L23 L24 L25 L26 | L1 L8 L9 L10 L11 L12 | L3 L14 L15 L16 L17 L18 | L1 L12 L19 L20 L21 L22 | L2 L4 L5 L6 L7 | L27 L28 L29 L30 bodies 1
extrude "Extrude4" add 1 faces at (33.6667, 11, 1) along direction (0, 0, 1) blind 3 on bodies 1 bodies 1
extrude "Extrude5" add sketch "Sketch1" against normal blind 1 contours L22 L23 L24 L25 bodies 1
sketch "Sketch4" plane through (0, 0, 0) normal (0, 0, -1) x (1, 0, 0)
  line L0 (8, 18) -> (43, 18)
  line L1 (43, 18) -> (43, -33)
  line L2 (43, -33) -> (8, -33)
  line L3 (8, -33) -> (8, 18)
  line L4 (50, -45.3866) -> (50, -33)
  line L5 (50, -33) -> (73.2304, -33)
  line L6 (73.2304, -33) -> (73.2304, -45.3866)
  line L7 (73.2304, -45.3866) -> (50, -45.3866)
  line L8 (1, -45.3866) -> (-19.7696, -45.3866)
  line L9 (-19.7696, -45.3866) -> (-19.7696, -25)
  line L10 (-19.7696, -25) -> (1, -25)
  line L11 (1, -25) -> (1, -45.3866)
  line L12 (1, -18) -> (-19.7696, -18)
  line L13 (-19.7696, -18) -> (-19.7696, 11)
  line L14 (-19.7696, 11) -> (1, 11)
  line L15 (1, 11) -> (1, -18)
  line L16 (1, 18) -> (-19.7696, 18)
  line L17 (-19.7696, 18) -> (-19.7696, 30.587)
  line L18 (-19.7696, 30.587) -> (1, 30.587)
  line L19 (1, 30.587) -> (1, 18)
  line L20 (50, 18) -> (50, 30.587)
  line L21 (50, 30.587) -> (73.2304, 30.587)
  line L22 (73.2304, 30.587) -> (73.2304, 18)
  line L23 (73.2304, 18) -> (50, 18)
  circle A0 centre (66.7314, 34.1104) radius 1.5
  circle A1 centre (-13.2624, -48.8983) radius 1.5
  circle A2 centre (-13.2753, 34.1171) radius 1.5
  circle A3 centre (66.7239, -48.8933) radius 1.5
  line L24 (50, 11) -> (73.2304, 11)
  line L25 (73.2304, 11) -> (73.2304, -26)
  line L26 (73.2304, -26) -> (50, -26)
  line L27 (50, -26) -> (50, 11)
  arc A4 (42.4985, 22.2168) -> (42.18, 25.4858) centre (42.4985, 23.8668) ccw
  line L28 (42.4985, 22.2168) -> (35.9985, 22.2168)
  line L29 (35.9985, 22.2168) -> (13.2, 21.981)
  line L30 (13.2, 21.981) -> (7.0185, 21.981)
  arc A5 (6.7, 25.25) -> (7.0185, 21.981) centre (6.7, 23.6) ccw
  line L31 (6.7, 25.25) -> (13.2, 25.25)
  line L32 (13.2, 25.25) -> (35.9985, 25.4858)
  line L33 (35.9985, 25.4858) -> (42.18, 25.4858)
  circle A6 centre (15.5775, -40.6826) radius 3.5
  circle A7 centre (33.2439, -40.7427) radius 3.5
  circle A8 centre (66.7314, 34.1104) radius 2.5
  circle A9 centre (-13.2753, 34.1171) radius 2.5
  circle A10 centre (-13.2624, -48.8983) radius 2.5
  circle A11 centre (66.7239, -48.8933) radius 2.5
  line L34 (80.2313, 37.6134) -> (-26.7696, 37.6134)
  line L35 (-26.7696, 37.6134) -> (-26.7696, -52.3866)
  line L36 (-26.7696, -52.3866) -> (80.2313, -52.3866)
  line L37 (80.2313, -52.3866) -> (80.2313, 37.6134)
  dimension "d43" = 5
  dimension "d44" = 5
  dimension "d45" = 5
  dimension "d46" = 5
  constraint concentric A0 A8
  constraint concentric A2 A9
  constraint concentric A1 A10
  constraint concentric A3 A11
  measures "d43" diameter of A8
  measures "d44" diameter of A9
  measures "d45" diameter of A10
  measures "d46" diameter of A11
fillet "Fillet1" radius 1 4 edges at (80.2313, 52.3866, 2) (-26.7696, 52.3866, 2) (-26.7696, -37.6134, 2) (80.2313, -37.6134, 2) on bodies 1
sketch "Sketch5" plane through (0, 0, -3) normal (0, 0, -1) x (1, 0, 0)
  line L0 (7.0185, 21.981) -> (13.2, 21.981)
  line L1 (13.2, 21.981) -> (13.2, 25.25)
  line L2 (13.2, 25.25) -> (6.7, 25.25)
  arc A0 (6.7, 25.25) -> (7.0185, 21.981) centre (6.7, 23.6) ccw
  line L3 (9.3739, 21.981) -> (9.3739, 25.25) construction
  circle A1 centre (9.3739, 23.6155) radius 1.375
  line L4 (42.18, 25.4858) -> (35.9985, 25.4858) construction
  line L5 (35.9985, 22.2168) -> (42.4985, 22.2168) construction
  line L6 (39.5332, 25.4858) -> (39.5332, 22.2168) construction
  circle A2 centre (39.5332, 23.8513) radius 1.375
  dimension "d56" = 2.75
  dimension "d57" = 2.75
  constraint coincident L0 L3.start
  constraint coincident L2 L3.end
  constraint perpendicular L2 L3
  constraint midpoint L3 A1.centre
  constraint coincident L4 L6.start
  constraint coincident L5 L6.end
  constraint perpendicular L5 L6
  constraint midpoint L6 A2.centre
  measures "d56" diameter of A1
  measures "d57" diameter of A2
extrude "Extrude7" cut sketch "Sketch5" against normal through all contours A1 | A2 bodies 1
sketch "Sketch6" plane through (0, 0, 4) normal (0, 0, 1) x (-1, 0, 0)
  circle A0 centre (-9.3739, 23.6155) radius 1.375
  circle A1 centre (-39.5332, 23.8513) radius 1.375
  line L0 (-50, 11) -> (-50, -26)
  line L1 (-50, -26) -> (-73.2304, -26)
  line L2 (-73.2304, -26) -> (-73.2304, 11)
  line L3 (-73.2304, 11) -> (-50, 11)
  line L4 (-50, -33) -> (-50, -45.3866)
  line L5 (-50, -45.3866) -> (-73.2304, -45.3866)
  line L6 (-73.2304, -45.3866) -> (-73.2304, -33)
  line L7 (-73.2304, -33) -> (-50, -33)
  line L8 (-1, -45.3866) -> (-1, -25)
  line L9 (-1, -25) -> (19.7696, -25)
  line L10 (19.7696, -25) -> (19.7696, -45.3866)
  line L11 (19.7696, -45.3866) -> (-1, -45.3866)
  line L12 (-1, -18) -> (-1, 11)
  line L13 (-1, 11) -> (19.7696, 11)
  line L14 (19.7696, 11) -> (19.7696, -18)
  line L15 (19.7696, -18) -> (-1, -18)
  line L16 (-1, 18) -> (-1, 30.587)
  line L17 (-1, 30.587) -> (19.7696, 30.587)
  line L18 (19.7696, 30.587) -> (19.7696, 18)
  line L19 (19.7696, 18) -> (-1, 18)
  arc A2 (-79.2313, 37.6134) -> (-80.2313, 36.6134) centre (-79.2313, 36.6134) ccw
  line L20 (-80.2313, 36.6134) -> (-80.2313, -51.3866)
  arc A3 (-80.2313, -51.3866) -> (-79.2313, -52.3866) centre (-79.2313, -51.3866) ccw
  line L21 (-79.2313, -52.3866) -> (25.7696, -52.3866)
  arc A4 (25.7696, -52.3866) -> (26.7696, -51.3866) centre (25.7696, -51.3866) ccw
  line L22 (26.7696, -51.3866) -> (26.7696, 36.6134)
  arc A5 (26.7696, 36.6134) -> (25.7696, 37.6134) centre (25.7696, 36.6134) ccw
  line L23 (25.7696, 37.6134) -> (-79.2313, 37.6134)
  circle A6 centre (-66.7314, 34.1104) radius 1.5
  circle A7 centre (13.2753, 34.1171) radius 1.5
  circle A8 centre (13.2624, -48.8983) radius 1.5
  circle A9 centre (-66.7239, -48.8933) radius 1.5
  line L24 (-50, 18) -> (-73.2304, 18)
  line L25 (-73.2304, 18) -> (-73.2304, 30.587)
  line L26 (-73.2304, 30.587) -> (-50, 30.587)
  line L27 (-50, 30.587) -> (-50, 18)
  line L28 (-35.9985, 22.2168) -> (-35.9985, 25.4858)
  line L29 (-35.9985, 25.4858) -> (-13.2, 25.25)
  line L30 (-13.2, 25.25) -> (-13.2, 21.981)
  line L31 (-13.2, 21.981) -> (-35.9985, 22.2168)
  line L32 (-36.9332, 25.3524) -> (-39.5332, 26.8536)
  line L33 (-39.5332, 26.8536) -> (-42.1332, 25.3524)
  line L34 (-42.1332, 25.3524) -> (-42.1332, 22.3502)
  line L35 (-42.1332, 22.3502) -> (-39.5332, 20.8491)
  line L36 (-39.5332, 20.8491) -> (-36.9332, 22.3502)
  line L37 (-36.9332, 22.3502) -> (-36.9332, 25.3524)
  line L38 (-6.7825, 25.1314) -> (-9.3909, 26.6177)
  line L39 (-9.3909, 26.6177) -> (-11.9824, 25.1018)
  line L40 (-11.9824, 25.1018) -> (-11.9653, 22.0997)
  line L41 (-11.9653, 22.0997) -> (-9.3568, 20.6133)
  line L42 (-9.3568, 20.6133) -> (-6.7654, 22.1292)
  line L43 (-6.7654, 22.1292) -> (-6.7825, 25.1314)
  point P0 (-39.5332, 23.8513)
  point P1 (-9.3739, 23.6155)
  dimension "d59" = 2.6
  dimension "d60" = 2.6
  constraint coincident P0 A1.centre
  constraint coincident A0.centre P1
  measures "d59" distance of P0 L37
  measures "d60" distance of P1 L43
extrude "Extrude8" cut sketch "Sketch6" against normal blind 1.85 contours L32 L33 L34 L35 L36 L37 | L38 L39 L40 L41 L42 L43 bodies 1
sketch "Sketch7" plane through (0, 0, -3) normal (0, 0, -1) x (1, 0, 0)
  circle A0 centre (33.2439, -40.7427) radius 3.5
  circle A1 centre (33.2439, -40.7427) radius 1.6
  circle A2 centre (15.5775, -40.6826) radius 1.6
  circle A3 centre (15.5775, -40.6826) radius 3.5
  dimension "d63" = 3.2
  dimension "d64" = 3.2
  constraint concentric A0 A1
  constraint concentric A2 A3
  measures "d63" diameter of A1
  measures "d64" diameter of A2
extrude "Extrude9" cut sketch "Sketch7" against normal through all contours A1 | A2 bodies 1